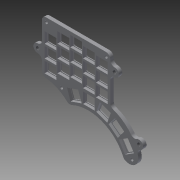
# Autodesk Inventor part: 20kb rebuild Printable Right
Saved by Autodesk Inventor 2015 SP2 (Build 190223200, 223)
## iProperties
Created: 2016-01-05
Part Number: 20kb rebuild Printable Right
Material: Generic
Document SubType Name: Modeling
Designer: Josh
Density: 1 g/cm^3
Appearance: Default
Author: Josh
Autodesk Inventor part; units mm, degrees
(part 1 of 2)
ref_plane "YZ Plane" through (0, 0, 0) normal (1, 0, 0) x (0, 1, 0)
ref_plane "XZ Plane" through (0, 0, 0) normal (0, 1, 0) x (-1, 0, 0)
ref_plane "XY Plane" through (0, 0, 0) normal (0, 0, 1) x (1, 0, 0)
sketch "Sketch1" plane through (0, 0, 0) normal (0, 0, 1) x (1, 0, 0)
  line L0 (0, 0) -> (19.05, 0)
  line L1 (19.05, 0) -> (19.05, 19.05)
  line L2 (19.05, 19.05) -> (0, 19.05)
  line L3 (0, 19.05) -> (0, 0)
  line L4 (19.05, 13.154) -> (19.05, 0)
  line L5 (19.05, 9.525) -> (38.1, 9.525)
  line L6 (38.1, 9.525) -> (38.1, 28.575)
  line L7 (38.1, 28.575) -> (19.05, 28.575)
  line L8 (19.05, 28.575) -> (19.05, 9.525)
  line L9 (38.1, 14.2875) -> (57.15, 14.2875)
  line L10 (57.15, 14.2875) -> (57.15, 33.3375)
  line L11 (57.15, 33.3375) -> (38.1, 33.3375)
  line L12 (38.1, 33.3375) -> (38.1, 14.2875)
  line L13 (57.15, 28.575) -> (76.2, 28.575)
  line L14 (76.2, 28.575) -> (76.2, 9.525)
  line L15 (76.2, 9.525) -> (57.15, 9.525)
  line L16 (57.15, 9.525) -> (57.15, 28.575)
  line L17 (76.2, 26.1938) -> (95.25, 26.1938)
  line L18 (95.25, 26.1938) -> (95.25, 7.1437)
  line L19 (95.25, 7.1437) -> (76.2, 7.1437)
  line L20 (76.2, 7.1437) -> (76.2, 26.1938)
  line L21 (19.05, 0) -> (21.4312, 0)
  line L22 (21.4312, 0) -> (21.4312, 9.525)
  line L23 (21.4312, 9.525) -> (19.05, 9.525)
  line L24 (19.05, 9.525) -> (19.05, 0)
  line L25 (38.1, 9.525) -> (40.4812, 9.525)
  line L26 (40.4812, 9.525) -> (40.4812, 14.2875)
  line L27 (40.4812, 14.2875) -> (38.1, 14.2875)
  line L28 (38.1, 14.2875) -> (38.1, 9.525)
  line L29 (57.15, 9.525) -> (54.7688, 9.525)
  line L30 (54.7688, 9.525) -> (54.7688, 14.2875)
  line L31 (54.7688, 14.2875) -> (57.15, 14.2875)
  line L32 (57.15, 14.2875) -> (57.15, 9.525)
  line L33 (76.2, 7.1437) -> (73.8187, 7.1438)
  line L34 (73.8187, 7.1438) -> (73.8187, 9.525)
  line L35 (73.8187, 9.525) -> (76.2, 9.525)
  line L36 (76.2, 9.525) -> (76.2, 7.1437)
  line L37 (39.1583, -17.1091) -> (57.15, -10.8479)
  line L38 (57.15, -10.8479) -> (50.8888, 7.1438)
  line L39 (50.8888, 7.1438) -> (32.8971, 0.8826)
  line L40 (32.8971, 0.8826) -> (39.1583, -17.1091)
  line L41 (57.15, -10.8479) -> (76.2, -10.8479)
  line L42 (76.2, -10.8479) -> (76.2, 8.2021)
  line L43 (76.2, 8.2021) -> (57.15, 8.2021)
  line L44 (57.15, 8.2021) -> (57.15, -10.8479)
  line L45 (76.2, -10.8479) -> (94.1917, -17.1091)
  line L46 (94.1917, -17.1091) -> (100.4529, 0.8826)
  line L47 (100.4529, 0.8826) -> (82.4612, 7.1437)
  line L48 (82.4612, 7.1437) -> (76.2, -10.8479)
  line L49 (94.1917, -17.1091) -> (109.1259, -28.9358)
  line L50 (109.1259, -28.9358) -> (120.9526, -14.0015)
  line L51 (120.9526, -14.0015) -> (106.0183, -2.1748)
  line L52 (106.0183, -2.1748) -> (94.1917, -17.1091)
  line L53 (109.1259, -28.9358) -> (119.3434, -45.0139)
  line L54 (119.3434, -45.0139) -> (135.4215, -34.7964)
  line L55 (135.4215, -34.7964) -> (125.204, -18.7183)
  line L56 (125.204, -18.7183) -> (109.1259, -28.9358)
  arc A0 (119.3434, -45.0139) -> (39.1583, -17.1091) centre (66.675, -67.1986) ccw
  line L57 (0, 19.05) -> (19.05, 19.05)
  line L58 (19.05, 19.05) -> (19.05, 38.1)
  line L59 (19.05, 38.1) -> (0, 38.1)
  line L60 (0, 38.1) -> (0, 19.05)
  line L61 (19.05, 28.575) -> (38.1, 28.575)
  line L62 (38.1, 28.575) -> (38.1, 47.625)
  line L63 (38.1, 47.625) -> (19.05, 47.625)
  line L64 (19.05, 47.625) -> (19.05, 28.575)
  line L65 (38.1, 33.3375) -> (57.15, 33.3375)
  line L66 (57.15, 33.3375) -> (57.15, 52.3875)
  line L67 (57.15, 52.3875) -> (38.1, 52.3875)
  line L68 (38.1, 52.3875) -> (38.1, 33.3375)
  line L69 (57.15, 47.625) -> (76.2, 47.625)
  line L70 (76.2, 47.625) -> (76.2, 28.575)
  line L71 (76.2, 28.575) -> (57.15, 28.575)
  line L72 (76.2, 45.2437) -> (95.25, 45.2437)
  line L73 (95.25, 45.2437) -> (95.25, 26.1937)
  line L74 (95.25, 26.1937) -> (76.2, 26.1937)
  line L75 (76.2, 26.1937) -> (76.2, 45.2437)
  line L76 (57.15, 33.3375) -> (57.15, 28.575)
  line L77 (0, 38.1) -> (19.05, 38.1)
  line L78 (19.05, 38.1) -> (19.05, 57.15)
  line L79 (19.05, 57.15) -> (0, 57.15)
  line L80 (0, 57.15) -> (0, 38.1)
  line L81 (19.05, 47.625) -> (38.1, 47.625)
  line L82 (38.1, 47.625) -> (38.1, 66.675)
  line L83 (38.1, 66.675) -> (19.05, 66.675)
  line L84 (19.05, 66.675) -> (19.05, 47.625)
  line L85 (38.1, 52.3875) -> (57.15, 52.3875)
  line L86 (57.15, 52.3875) -> (57.15, 71.4375)
  line L87 (57.15, 71.4375) -> (38.1, 71.4375)
  line L88 (38.1, 71.4375) -> (38.1, 52.3875)
  line L89 (57.15, 66.675) -> (76.2, 66.675)
  line L90 (76.2, 66.675) -> (76.2, 47.625)
  line L91 (76.2, 47.625) -> (57.15, 47.625)
  line L92 (76.2, 64.2938) -> (95.25, 64.2938)
  line L93 (95.25, 64.2938) -> (95.25, 45.2437)
  line L94 (95.25, 45.2437) -> (76.2, 45.2437)
  line L95 (76.2, 45.2437) -> (76.2, 64.2938)
  line L96 (57.15, 52.3875) -> (57.15, 47.625)
  line L97 (0, 71.4375) -> (9.525, 71.4375)
  line L98 (9.525, 71.4375) -> (9.525, 61.9125)
  line L99 (9.525, 61.9125) -> (0, 61.9125)
  line L100 (0, 61.9125) -> (0, 71.4375)
  line L101 (83.31, 61.9125) -> (92.835, 61.9125)
  line L102 (92.835, 61.9125) -> (92.835, 71.4375)
  line L103 (92.835, 71.4375) -> (83.31, 71.4375)
  line L104 (83.31, 71.4375) -> (83.31, 61.9125)
  line L105 (9.525, 55.5625) -> (19.05, 55.5625)
  line L106 (19.05, 55.5625) -> (19.05, 71.4375)
  line L107 (19.05, 71.4375) -> (9.525, 71.4375)
  line L108 (9.525, 71.4375) -> (9.525, 55.5625)
  circle A1 centre (7.1852, 59.8202) radius 2.0923
  line L109 (53.975, 71.4375) -> (57.15, 71.4375)
  line L110 (57.15, 71.4375) -> (57.15, 74.6125)
  line L111 (57.15, 74.6125) -> (53.975, 74.6125)
  line L112 (53.975, 74.6125) -> (53.975, 71.4375)
  line L113 (0, 0) -> (-3.175, 0)
  line L114 (-3.175, 0) -> (-3.175, -3.175)
  line L115 (-3.175, -3.175) -> (0, -3.175)
  line L116 (0, -3.175) -> (0, 0)
  line L117 (95.25, 7.1437) -> (98.425, 7.1437)
  line L118 (98.425, 7.1437) -> (98.425, 10.3187)
  line L119 (98.425, 10.3187) -> (95.25, 10.3187)
  line L120 (95.25, 10.3187) -> (95.25, 7.1437)
  line L121 (95.25, 64.2938) -> (98.425, 64.2938)
  line L122 (98.425, 64.2938) -> (98.425, 67.4688)
  line L123 (98.425, 67.4688) -> (95.25, 67.4688)
  line L124 (95.25, 67.4688) -> (95.25, 64.2938)
  line L125 (-3.175, -3.175) -> (-3.175, 74.6125)
  line L126 (-3.175, 74.6125) -> (98.425, 74.6125)
  line L127 (98.425, 74.6125) -> (98.425, 7.1437)
  line L128 (40.2019, -20.1077) -> (39.1583, -17.1091)
  line L129 (39.1583, -17.1091) -> (36.1597, -18.1526)
  line L130 (36.1597, -18.1526) -> (37.2033, -21.1512)
  line L131 (37.2033, -21.1512) -> (40.2019, -20.1077)
  line L132 (40.2019, -20.1077) -> (36.1597, -18.1526) construction
  line L133 (39.1583, -17.1091) -> (37.2033, -21.1512) construction
  line L134 (116.6637, -46.7168) -> (118.3666, -49.3965)
  line L135 (118.3666, -49.3965) -> (121.0463, -47.6936)
  line L136 (121.0463, -47.6936) -> (119.3434, -45.0139)
  line L137 (119.3434, -45.0139) -> (116.6637, -46.7168)
  line L138 (116.6637, -46.7168) -> (121.0463, -47.6936) construction
  line L139 (118.3666, -49.3965) -> (119.3434, -45.0139) construction
  line L140 (135.4215, -34.7964) -> (137.1244, -37.4761)
  line L141 (137.1244, -37.4761) -> (139.8041, -35.7732)
  line L142 (139.8041, -35.7732) -> (138.1012, -33.0935)
  line L143 (138.1012, -33.0935) -> (135.4215, -34.7964)
  line L144 (135.4215, -34.7964) -> (139.8041, -35.7732) construction
  line L145 (137.1244, -37.4761) -> (138.1012, -33.0935) construction
  arc A2 (37.2033, -21.1512) -> (-3.175, -3.175) centre (-3.175, -57.512) ccw
  arc A3 (118.3666, -49.3965) -> (37.2033, -21.1512) centre (65.4005, -70.8608) ccw
  arc A4 (118.3666, -49.3965) -> (139.8041, -35.7732) centre (126.6171, -38.7007) ccw
  arc A5 (139.8041, -35.7732) -> (98.425, 7.1437) centre (84.0124, -48.1591) ccw
  point P0 (82.4612, 26.1937)
  point P1 (82.4612, 45.2437)
  point P2 (38.1808, -19.1302)
  point P3 (118.855, -47.2052)
  point P4 (137.6128, -35.2848)
  dimension "d0" = 19.05
  dimension "d1" = 9.525
  dimension "d2" = 4.7625
  dimension "d3" = 2.3813
  dimension "d4" = 57.15
  dimension "d7" = 19.05
  dimension "d12" = 9.525
  dimension "d13" = 9.525
  dimension "d14" = 15.875
  dimension "d15" = 3.175
  constraints: 292 end point, 48 parallel, 40 equal length, 25 perpendicular, 23 collinear, 17 horizontal, 14 point on circle, 6 centre point, 6 midpoint, 4 point on line, 3 tangent, 2 equal radius, 1 coincident, 1 vertical, 83 other
  measures "d0" distance of L2.end L1.end
  measures "d1" distance of L21.end L22.end
  measures "d2" distance of L25.end L26.end
  measures "d3" distance of L33.end L34.end
  measures "d4" radius of A0
  measures "d7" distance of L1.end L59.start
  measures "d12" distance of L98.end L99.end
  measures "d13" distance of L102.end L103.end
  measures "d14" distance of L97.end L105.start
  measures "d15" distance of L111.end L110.end
extrude "Extrusion1" add sketch "Sketch1" along normal blind 5.08 contours L3 L2 L1 L0 | A1 | L113 L125 L126 L112 L87 L88 L83 L106 L107 L97 L100 L99 L108 L79 L80 L60 L3 | L116 L115 L114 L113 | L0 L21 L22 L5 L25 L26 L9 L30 L29 L15 L34 L43 L44 L38 L39 L40 L129 L130 A2 L115 L116 | L1 L5 L22 L21 | L60 L59 L58 L8 L2 | L1 L8 L7 L6 L5 | L80 L79 L108 L105 L78 L64 L59 | L58 L64 L63 L62 L12 L7 | L130 L129 L128 A3 | L111 L110 L87 L112 | L6 L9 L26 L25 | L12 L11 L10 L9 L6 | L78 L84 L83 L82 L68 L63 | L108 L98 L107 L106 L84 L79 | L79 L78 L105 L108 | L128 L37 L41 L45 L49 L53 L137 A3 | L126 L127 L123 L124 L92 L102 L103 L104 L90 L89 L86 L110 | L87 L86 L67 L82 L88 | L62 L68 L67 L66 L11 | L99 L100 L97 L98 | A0 L37 | L40 L39 L38 A0 | L137 L136 L135 A3 | L66 L69 L70 L13 L10 | A0 L41 | L44 L43 L34 L33 L42 A0 | A0 L56 L55 L54 | L53 A0 | L54 L140 L141 A4 L135 L136 | L89 L90 L69 L66 L86 | L122 L121 L124 L123 | L9 L16 L29 L30 | L13 L14 L15 L16 L10 | A0 L45 | L42 L19 L48 | L48 L47 L46 A0 | A0 L52 L51 L50 | L50 L51 L52 L46 L47 L19 L117 A5 L142 L143 L55 L56 | L49 A0 | L143 L142 L141 L140 | L127 L119 L18 L73 L93 L121 | L70 L72 L73 L17 L14 | L90 L92 L104 L101 L102 L93 L72 L70 | L20 L14 L17 L18 L19 | L33 L34 L43 L20 | L34 L15 L20 L43 | L117 L18 L119 L118 | L104 L103 L102 L92 | L92 L102 L101 L104
sketch "Sketch2" plane through (0, 0, 5.08) normal (0, 0, 1) x (1, 0, 0)
  line L0 (0, 0) -> (19.05, 0) projected
  line L1 (0, 19.05) -> (0, 0) projected
  line L2 (19.05, 19.05) -> (0, 19.05) projected
  line L3 (19.05, 0) -> (19.05, 19.05) projected
  line L4 (19.05, 9.525) -> (38.1, 9.525) projected
  line L5 (19.05, 28.575) -> (19.05, 9.525) projected
  line L6 (38.1, 9.525) -> (38.1, 28.575) projected
  line L7 (38.1, 28.575) -> (19.05, 28.575) projected
  line L8 (38.1, 14.2875) -> (57.15, 14.2875) projected
  line L9 (57.15, 33.3375) -> (38.1, 33.3375) projected
  line L10 (57.15, 14.2875) -> (57.15, 33.3375) projected
  line L11 (57.15, 28.575) -> (76.2, 28.575) projected
  line L12 (76.2, 9.525) -> (57.15, 9.525) projected
  line L13 (76.2, 26.1938) -> (95.25, 26.1938) projected
  line L14 (95.25, 26.1938) -> (95.25, 7.1437) projected
  line L15 (95.25, 7.1437) -> (76.2, 7.1437) projected
  line L16 (76.2, 28.575) -> (76.2, 9.525) projected
  line L17 (38.1, 33.3375) -> (38.1, 14.2875) projected
  line L18 (57.15, 9.525) -> (57.15, 28.575) projected
  line L19 (76.2, 7.1437) -> (76.2, 26.1938) projected
  line L20 (19.05, 19.05) -> (0, 0) construction
  line L21 (0, 19.05) -> (19.05, 0) construction
  line L22 (19.05, 28.575) -> (38.1, 9.525) construction
  line L23 (38.1, 28.575) -> (19.05, 9.525) construction
  line L24 (38.1, 33.3375) -> (57.15, 14.2875) construction
  line L25 (57.15, 33.3375) -> (38.1, 14.2875) construction
  line L26 (57.15, 28.575) -> (76.2, 9.525) construction
  line L27 (76.2, 28.575) -> (57.15, 9.525) construction
  line L28 (76.2, 26.1938) -> (95.25, 7.1437) construction
  line L29 (76.2, 7.1437) -> (95.25, 26.1938) construction
  line L30 (2.525, 2.525) -> (16.525, 2.525)
  line L31 (16.525, 2.525) -> (16.525, 16.525)
  line L32 (16.525, 16.525) -> (2.525, 16.525)
  line L33 (2.525, 16.525) -> (2.525, 2.525)
  line L34 (2.525, 2.525) -> (16.525, 16.525) construction
  line L35 (16.525, 2.525) -> (2.525, 16.525) construction
  line L36 (21.575, 12.05) -> (35.575, 12.05)
  line L37 (35.575, 12.05) -> (35.575, 26.05)
  line L38 (35.575, 26.05) -> (21.575, 26.05)
  line L39 (21.575, 26.05) -> (21.575, 12.05)
  line L40 (21.575, 12.05) -> (35.575, 26.05) construction
  line L41 (35.575, 12.05) -> (21.575, 26.05) construction
  line L42 (40.625, 16.8125) -> (54.625, 16.8125)
  line L43 (54.625, 16.8125) -> (54.625, 30.8125)
  line L44 (54.625, 30.8125) -> (40.625, 30.8125)
  line L45 (40.625, 30.8125) -> (40.625, 16.8125)
  line L46 (40.625, 16.8125) -> (54.625, 30.8125) construction
  line L47 (54.625, 16.8125) -> (40.625, 30.8125) construction
  line L48 (59.675, 12.05) -> (73.675, 12.05)
  line L49 (73.675, 12.05) -> (73.675, 26.05)
  line L50 (73.675, 26.05) -> (59.675, 26.05)
  line L51 (59.675, 26.05) -> (59.675, 12.05)
  line L52 (59.675, 12.05) -> (73.675, 26.05) construction
  line L53 (73.675, 12.05) -> (59.675, 26.05) construction
  line L54 (78.725, 9.6688) -> (92.725, 9.6688)
  line L55 (92.725, 9.6688) -> (92.725, 23.6688)
  line L56 (92.725, 23.6688) -> (78.725, 23.6688)
  line L57 (78.725, 23.6688) -> (78.725, 9.6688)
  line L58 (78.725, 9.6688) -> (92.725, 23.6688) construction
  line L59 (92.725, 9.6688) -> (78.725, 23.6688) construction
  line L60 (1.775, 3.125) -> (17.275, 3.125)
  line L61 (17.275, 3.125) -> (17.275, 15.925)
  line L62 (17.275, 15.925) -> (1.775, 15.925)
  line L63 (1.775, 15.925) -> (1.775, 3.125)
  line L64 (1.775, 3.125) -> (17.275, 15.925) construction
  line L65 (17.275, 3.125) -> (1.775, 15.925) construction
  line L66 (20.825, 12.65) -> (36.325, 12.65)
  line L67 (36.325, 12.65) -> (36.325, 25.45)
  line L68 (36.325, 25.45) -> (20.825, 25.45)
  line L69 (20.825, 25.45) -> (20.825, 12.65)
  line L70 (20.825, 12.65) -> (36.325, 25.45) construction
  line L71 (36.325, 12.65) -> (20.825, 25.45) construction
  line L72 (39.875, 17.4125) -> (55.375, 17.4125)
  line L73 (55.375, 17.4125) -> (55.375, 30.2125)
  line L74 (55.375, 30.2125) -> (39.875, 30.2125)
  line L75 (39.875, 30.2125) -> (39.875, 17.4125)
  line L76 (39.875, 17.4125) -> (55.375, 30.2125) construction
  line L77 (55.375, 17.4125) -> (39.875, 30.2125) construction
  line L78 (58.925, 12.65) -> (74.425, 12.65)
  line L79 (74.425, 12.65) -> (74.425, 25.45)
  line L80 (74.425, 25.45) -> (58.925, 25.45)
  line L81 (58.925, 25.45) -> (58.925, 12.65)
  line L82 (58.925, 12.65) -> (74.425, 25.45) construction
  line L83 (74.425, 12.65) -> (58.925, 25.45) construction
  line L84 (77.975, 10.2688) -> (93.475, 10.2688)
  line L85 (93.475, 10.2688) -> (93.475, 23.0688)
  line L86 (93.475, 23.0688) -> (77.975, 23.0688)
  line L87 (77.975, 23.0688) -> (77.975, 10.2688)
  line L88 (77.975, 10.2688) -> (93.475, 23.0688) construction
  line L89 (93.475, 10.2688) -> (77.975, 23.0688) construction
  point P0 (9.525, 9.525)
  point P1 (28.575, 19.05)
  point P2 (47.625, 23.8125)
  point P3 (66.675, 19.05)
  point P4 (85.725, 16.6687)
  dimension "d18" = 14
  dimension "d19" = 15.5
  dimension "d20" = 12.8
  constraints: 140 end point, 26 midpoint, 21 parallel, 18 perpendicular, 17 equal length, 10 horizontal
  measures "d18" distance of L31.end L32.end
  measures "d19" distance of L61.end L62.end
  measures "d20" distance of L60.end L61.end
extrude "Extrusion2" cut sketch "Sketch2" against normal blind 5.08 contours L33 L60 L31 L30 | L60 L63 L62 L33 | L33 L62 L31 L60 | L31 L62 L61 L60 | L33 L32 L31 L62 | L39 L66 L37 L36 | L66 L69 L68 L39 | L39 L68 L37 L66 | L37 L68 L67 L66 | L39 L38 L37 L68 | L45 L72 L43 L42 | L72 L75 L74 L45 | L45 L74 L43 L72 | L43 L74 L73 L72 | L45 L44 L43 L74 | L51 L78 L49 L48 | L78 L81 L80 L51 | L51 L80 L49 L78 | L49 L80 L79 L78 | L51 L50 L49 L80 | L57 L84 L55 L54 | L84 L87 L86 L57 | L57 L86 L55 L84 | L55 L86 L85 L84 | L57 L56 L55 L86
sketch "Sketch3" plane through (0, 0, 5.08) normal (0, 0, 1) x (1, 0, 0)
  line L0 (0.775, 1.525) -> (18.275, 1.525)
  line L1 (18.275, 1.525) -> (18.275, 17.525)
  line L2 (18.275, 17.525) -> (0.775, 17.525)
  line L3 (0.775, 17.525) -> (0.775, 1.525)
  line L4 (0.775, 1.525) -> (18.275, 17.525) construction
  line L5 (18.275, 1.525) -> (0.775, 17.525) construction
  line L6 (19.825, 27.05) -> (37.325, 27.05)
  line L7 (37.325, 27.05) -> (37.325, 11.05)
  line L8 (37.325, 11.05) -> (19.825, 11.05)
  line L9 (19.825, 11.05) -> (19.825, 27.05)
  line L10 (19.825, 27.05) -> (37.325, 11.05) construction
  line L11 (37.325, 27.05) -> (19.825, 11.05) construction
  line L12 (38.875, 31.8125) -> (56.375, 31.8125)
  line L13 (56.375, 31.8125) -> (56.375, 15.8125)
  line L14 (56.375, 15.8125) -> (38.875, 15.8125)
  line L15 (38.875, 15.8125) -> (38.875, 31.8125)
  line L16 (38.875, 31.8125) -> (56.375, 15.8125) construction
  line L17 (56.375, 31.8125) -> (38.875, 15.8125) construction
  line L18 (75.425, 27.05) -> (57.925, 27.05)
  line L19 (57.925, 27.05) -> (57.925, 11.05)
  line L20 (57.925, 11.05) -> (75.425, 11.05)
  line L21 (75.425, 11.05) -> (75.425, 27.05)
  line L22 (75.425, 27.05) -> (57.925, 11.05) construction
  line L23 (57.925, 27.05) -> (75.425, 11.05) construction
  line L24 (76.975, 8.6687) -> (94.475, 8.6687)
  line L25 (94.475, 8.6687) -> (94.475, 24.6687)
  line L26 (94.475, 24.6687) -> (76.975, 24.6687)
  line L27 (76.975, 24.6687) -> (76.975, 8.6687)
  line L28 (76.975, 8.6687) -> (94.475, 24.6687) construction
  line L29 (94.475, 8.6687) -> (76.975, 24.6687) construction
  point P0 (0, 0)
  point P1 (9.525, 9.525)
  point P2 (28.575, 19.05)
  point P3 (47.625, 23.8125)
  point P4 (66.675, 19.05)
  point P5 (85.725, 16.6687)
  dimension "d23" = 17.5
  dimension "d24" = 16
  constraints: 60 end point, 17 parallel, 10 midpoint, 5 horizontal, 5 perpendicular, 1 point on line
  measures "d23" distance of L1.end L2.end
  measures "d24" distance of L0.end L1.end
extrude "Extrusion3" cut sketch "Sketch3" against normal blind 3.98
pattern_linear "Rectangular Pattern1" count 3 spacing 19.05 along (0, 1, 0) of "Extrusion2", "Extrusion3"
sketch "Sketch4" plane through (0, 0, 5.08) normal (0, 0, 1) x (1, 0, 0)
  line L0 (57.15, -10.8479) -> (50.8888, 7.1438) projected
  line L1 (39.1583, -17.1091) -> (57.15, -10.8479) projected
  line L2 (32.8971, 0.8826) -> (39.1583, -17.1091) projected
  line L3 (50.8888, 7.1438) -> (32.8971, 0.8826) projected
  line L4 (57.15, 8.2021) -> (57.15, -10.8479) projected
  line L5 (76.2, 8.2021) -> (57.15, 8.2021) projected
  line L6 (76.2, -10.8479) -> (76.2, 8.2021) projected
  line L7 (57.15, -10.8479) -> (76.2, -10.8479) projected
  line L8 (82.4612, 7.1437) -> (76.2, -10.8479) projected
  line L9 (100.4529, 0.8826) -> (82.4612, 7.1437) projected
  line L10 (94.1917, -17.1091) -> (100.4529, 0.8826) projected
  line L11 (76.2, -10.8479) -> (94.1917, -17.1091) projected
  line L12 (106.0183, -2.1748) -> (94.1917, -17.1091) projected
  line L13 (120.9526, -14.0015) -> (106.0183, -2.1748) projected
  line L14 (109.1259, -28.9358) -> (120.9526, -14.0015) projected
  line L15 (94.1917, -17.1091) -> (109.1259, -28.9358) projected
  line L16 (109.1259, -28.9358) -> (119.3434, -45.0139) projected
  line L17 (125.204, -18.7183) -> (109.1259, -28.9358) projected
  line L18 (135.4215, -34.7964) -> (125.204, -18.7183) projected
  line L19 (119.3434, -45.0139) -> (135.4215, -34.7964) projected
  line L20 (32.8971, 0.8826) -> (57.15, -10.8479) construction
  line L21 (50.8888, 7.1438) -> (39.1583, -17.1091) construction
  line L22 (57.15, 8.2021) -> (76.2, -10.8479) construction
  line L23 (76.2, 8.2021) -> (57.15, -10.8479) construction
  line L24 (82.4612, 7.1437) -> (94.1917, -17.1091) construction
  line L25 (76.2, -10.8479) -> (100.4529, 0.8826) construction
  line L26 (106.0183, -2.1748) -> (109.1259, -28.9358) construction
  line L27 (120.9526, -14.0015) -> (94.1917, -17.1091) construction
  line L28 (125.204, -18.7183) -> (119.3434, -45.0139) construction
  line L29 (109.1259, -28.9358) -> (135.4215, -34.7964) construction
  line L30 (-25.4225, -31.5333) -> (-11.4225, -31.5333) construction
  line L31 (-11.4225, -31.5333) -> (-11.4225, -17.5333) construction
  line L32 (-11.4225, -17.5333) -> (-25.4225, -17.5333) construction
  line L33 (-25.4225, -17.5333) -> (-25.4225, -31.5333) construction
  line L34 (-25.4225, -31.5333) -> (-11.4225, -17.5333) construction
  line L35 (-11.4225, -31.5333) -> (-25.4225, -17.5333) construction
  line L36 (-21.2907, -27.4015) -> (-15.5542, -27.4015) construction
  line L37 (-15.5542, -27.4015) -> (-15.5542, -21.6651) construction
  line L38 (-15.5542, -21.6651) -> (-21.2907, -21.6651) construction
  line L39 (-21.2907, -21.6651) -> (-21.2907, -27.4015) construction
  line L40 (-21.2907, -27.4015) -> (-15.5542, -21.6651) construction
  line L41 (-15.5542, -27.4015) -> (-21.2907, -21.6651) construction
  line L42 (79.4146, -9.2931) -> (92.6368, -13.8945)
  line L43 (92.6368, -13.8945) -> (97.2382, -0.6723)
  line L44 (97.2382, -0.6723) -> (84.016, 3.9291)
  line L45 (84.016, 3.9291) -> (79.4146, -9.2931)
  line L46 (79.4146, -9.2931) -> (97.2382, -0.6723) construction
  line L47 (92.6368, -13.8945) -> (84.016, 3.9291) construction
  line L48 (97.7387, -16.6972) -> (108.714, -25.3887)
  line L49 (108.714, -25.3887) -> (117.4056, -14.4134)
  line L50 (117.4056, -14.4134) -> (106.4302, -5.7219)
  line L51 (106.4302, -5.7219) -> (97.7387, -16.6972)
  line L52 (97.7387, -16.6972) -> (117.4056, -14.4134) construction
  line L53 (108.714, -25.3887) -> (106.4302, -5.7219) construction
  line L54 (112.6113, -29.7126) -> (120.1202, -41.5285)
  line L55 (120.1202, -41.5285) -> (131.9361, -34.0196)
  line L56 (131.9361, -34.0196) -> (124.4272, -22.2037)
  line L57 (124.4272, -22.2037) -> (112.6113, -29.7126)
  line L58 (112.6113, -29.7126) -> (131.9361, -34.0196) construction
  line L59 (120.1202, -41.5285) -> (124.4272, -22.2037) construction
  line L60 (40.7132, -13.8945) -> (53.9354, -9.2931)
  line L61 (53.9354, -9.2931) -> (49.334, 3.9291)
  line L62 (49.334, 3.9291) -> (36.1118, -0.6723)
  line L63 (36.1118, -0.6723) -> (40.7132, -13.8945)
  line L64 (40.7132, -13.8945) -> (49.334, 3.9291) construction
  line L65 (53.9354, -9.2931) -> (36.1118, -0.6723) construction
  line L66 (59.675, -8.3229) -> (73.675, -8.3229)
  line L67 (73.675, -8.3229) -> (73.675, 5.6771)
  line L68 (73.675, 5.6771) -> (59.675, 5.6771)
  line L69 (59.675, 5.6771) -> (59.675, -8.3229)
  line L70 (59.675, -8.3229) -> (73.675, 5.6771) construction
  line L71 (73.675, -8.3229) -> (59.675, 5.6771) construction
  line L72 (35.6006, -1.4854) -> (50.2395, 3.609)
  line L73 (50.2395, 3.609) -> (54.4465, -8.4799)
  line L74 (54.4465, -8.4799) -> (39.8076, -13.5743)
  line L75 (39.8076, -13.5743) -> (35.6006, -1.4854)
  line L76 (35.6006, -1.4854) -> (54.4465, -8.4799) construction
  line L77 (50.2395, 3.609) -> (39.8076, -13.5743) construction
  line L78 (58.925, -7.7229) -> (74.425, -7.7229)
  line L79 (74.425, -7.7229) -> (74.425, 5.0771)
  line L80 (74.425, 5.0771) -> (58.925, 5.0771)
  line L81 (58.925, 5.0771) -> (58.925, -7.7229)
  line L82 (58.925, -7.7229) -> (74.425, 5.0771) construction
  line L83 (74.425, -7.7229) -> (58.925, 5.0771) construction
  line L84 (121.0289, -41.8397) -> (112.7154, -28.7578)
  line L85 (112.7154, -28.7578) -> (123.5186, -21.8925)
  line L86 (123.5186, -21.8925) -> (131.832, -34.9744)
  line L87 (131.832, -34.9744) -> (121.0289, -41.8397)
  line L88 (121.0289, -41.8397) -> (123.5186, -21.8925) construction
  line L89 (112.7154, -28.7578) -> (131.832, -34.9744) construction
  line L90 (-26.1725, -18.1333) -> (-10.6725, -18.1333) construction
  line L91 (-10.6725, -18.1333) -> (-10.6725, -30.9333) construction
  line L92 (-10.6725, -30.9333) -> (-26.1725, -30.9333) construction
  line L93 (-26.1725, -30.9333) -> (-26.1725, -18.1333) construction
  line L94 (-26.1725, -18.1333) -> (-10.6725, -30.9333) construction
  line L95 (-10.6725, -18.1333) -> (-26.1725, -30.9333) construction
  line L96 (97.5233, -15.7612) -> (109.6745, -25.384)
  line L97 (109.6745, -25.384) -> (117.621, -15.3494)
  line L98 (117.621, -15.3494) -> (105.4698, -5.7266)
  line L99 (105.4698, -5.7266) -> (97.5233, -15.7612)
  line L100 (97.5233, -15.7612) -> (117.621, -15.3494) construction
  line L101 (109.6745, -25.384) -> (105.4698, -5.7266) construction
  line L102 (78.9035, -8.4799) -> (93.5424, -13.5743)
  line L103 (93.5424, -13.5743) -> (97.7494, -1.4854)
  line L104 (97.7494, -1.4854) -> (83.1105, 3.609)
  line L105 (83.1105, 3.609) -> (78.9035, -8.4799)
  line L106 (78.9035, -8.4799) -> (97.7494, -1.4854) construction
  line L107 (93.5424, -13.5743) -> (83.1105, 3.609) construction
  point P0 (0, 0)
  point P1 (-18.4225, -24.5333)
  point P2 (-18.4225, -24.5333)
  point P3 (88.3264, -4.9827)
  point P4 (107.5721, -15.5553)
  point P5 (122.2737, -31.8661)
  point P6 (45.0236, -4.9827)
  point P7 (66.675, -1.3229)
  dimension "d30" = 14
  dimension "d31" = 15.5
  dimension "d32" = 12.8
  constraints: 176 end point, 36 parallel, 32 midpoint, 21 equal length, 18 perpendicular, 3 horizontal, 1 point on line
  measures "d30" distance of L31.end L32.end
  measures "d31" distance of L90.start L90.end
  measures "d32" distance of L90.end L91.end
extrude "Extrusion4" cut sketch "Sketch4" against normal blind 5.08 contours L45 L102 L43 L42 | L102 L105 L104 L45 | L45 L104 L43 L102 | L43 L104 L103 L102 | L45 L44 L43 L104 | L51 L96 L49 L48 | L96 L99 L98 L51 | L51 L98 L49 L96 | L49 L98 L97 L96 | L51 L50 L49 L98 | L57 L84 L55 L54 | L84 L85 L86 L57 | L57 L86 L55 L84 | L55 L86 L87 L84 | L57 L56 L55 L86 | L63 L74 L61 L60 | L74 L75 L72 L63 | L63 L72 L61 L74 | L61 L72 L73 L74 | L63 L62 L61 L72 | L69 L78 L67 L66 | L78 L81 L80 L69 | L69 L80 L67 L78 | L67 L80 L79 L78 | L69 L68 L67 L80
sketch "Sketch5" plane through (0, 0, 5.08) normal (0, 0, 1) x (1, 0, 0)
  line L0 (18.275, 1.525) -> (0.775, 1.525) projected
  line L1 (18.275, 17.525) -> (18.275, 1.525) projected
  line L2 (0.775, 17.525) -> (18.275, 17.525) projected
  line L3 (0.775, 1.525) -> (0.775, 17.525) projected
  line L4 (53.9354, -9.2931) -> (40.7132, -13.8945) projected
  line L5 (73.675, -8.3229) -> (59.675, -8.3229) projected
  line L6 (92.6368, -13.8945) -> (79.4146, -9.2931) projected
  line L7 (108.714, -25.3887) -> (97.7387, -16.6972) projected
  line L8 (120.1202, -41.5285) -> (112.6113, -29.7126) projected
  line L9 (39.3891, -15.4141) -> (55.9168, -9.6624)
  line L10 (55.9168, -9.6624) -> (50.6581, 5.4488)
  line L11 (50.6581, 5.4488) -> (34.1303, -0.303)
  line L12 (34.1303, -0.303) -> (39.3891, -15.4141)
  line L13 (39.3891, -15.4141) -> (50.6581, 5.4488) construction
  line L14 (55.9168, -9.6624) -> (34.1303, -0.303) construction
  line L15 (57.925, -9.3229) -> (75.425, -9.3229)
  line L16 (75.425, -9.3229) -> (75.425, 6.6771)
  line L17 (75.425, 6.6771) -> (57.925, 6.6771)
  line L18 (57.925, 6.6771) -> (57.925, -9.3229)
  line L19 (57.925, -9.3229) -> (75.425, 6.6771) construction
  line L20 (75.425, -9.3229) -> (57.925, 6.6771) construction
  line L21 (77.4332, -9.6624) -> (93.9609, -15.4141)
  line L22 (93.9609, -15.4141) -> (99.2197, -0.303)
  line L23 (99.2197, -0.303) -> (82.6919, 5.4488)
  line L24 (82.6919, 5.4488) -> (77.4332, -9.6624)
  line L25 (77.4332, -9.6624) -> (99.2197, -0.303) construction
  line L26 (93.9609, -15.4141) -> (82.6919, 5.4488) construction
  line L27 (109.4651, -27.2591) -> (95.746, -16.3947)
  line L28 (95.746, -16.3947) -> (105.6792, -3.8515)
  line L29 (105.6792, -3.8515) -> (119.3983, -14.7159)
  line L30 (119.3983, -14.7159) -> (109.4651, -27.2591)
  line L31 (109.4651, -27.2591) -> (105.6792, -3.8515) construction
  line L32 (95.746, -16.3947) -> (119.3983, -14.7159) construction
  line L33 (120.2148, -43.5419) -> (110.8287, -28.7719)
  line L34 (110.8287, -28.7719) -> (124.3326, -20.1903)
  line L35 (124.3326, -20.1903) -> (133.7188, -34.9602)
  line L36 (133.7188, -34.9602) -> (120.2148, -43.5419)
  line L37 (120.2148, -43.5419) -> (124.3326, -20.1903) construction
  line L38 (110.8287, -28.7719) -> (133.7188, -34.9602) construction
  point P0 (0, 0)
  point P1 (45.0236, -4.9827)
  point P2 (66.675, -1.3229)
  point P3 (88.3264, -4.9827)
  point P4 (107.5721, -15.5553)
  point P5 (122.2737, -31.8661)
  constraints: 60 end point, 15 parallel, 10 equal length, 10 midpoint, 5 perpendicular
extrude "Extrusion5" cut sketch "Sketch5" against normal blind 3.98 contours L12 L11 L10 L9 | L18 L17 L16 L15 | L24 L23 L22 L21 | L27 L28 L29 L30 | L33 L34 L35 L36
fillet "Fillet1" radius 6.35 6 edges at (37.2033, -21.1512, 2.54) (-3.175, -3.175, 2.54) (98.425, 7.1438, 2.54) (98.425, 74.6125, 2.54) (-3.175, 74.6125, 2.54) (118.3666, -49.3965, 2.54)
sketch "Sketch6" plane through (0, 0, 0) normal (0, 0, -1) x (-1, 0, 0)
  line L0 (-37.9981, 73.8371) -> (-5.6484, 73.8371) construction
  line L1 (-5.6484, 73.8371) -> (-5.6484, 68.2625) construction
  line L2 (-5.6484, 68.2625) -> (-37.9981, 68.2625) construction
  line L3 (-37.9981, 68.2625) -> (-37.9981, 73.8371) construction
  line L4 (-89.6016, 73.8371) -> (-70.2241, 73.8371) construction
  line L5 (-70.2241, 73.8371) -> (-70.2241, 68.2625) construction
  line L6 (-70.2241, 68.2625) -> (-89.6016, 68.2625) construction
  line L7 (-89.6016, 68.2625) -> (-89.6016, 73.8371) construction
  line L8 (-114.209, 73.8371) -> (51.1131, 73.8371) construction
  line L9 (-70.2241, 68.2625) -> (-37.9981, 68.2625) construction
  line L10 (-37.9981, 68.2625) -> (-37.9981, 73.8371) construction
  line L11 (-37.9981, 73.8371) -> (-70.2241, 73.8371) construction
  line L12 (-70.2241, 73.8371) -> (-70.2241, 68.2625) construction
  arc A0 (-92.075, 74.6125) -> (-98.425, 68.2625) centre (-92.075, 68.2625) ccw construction
  arc A1 (3.175, 68.2625) -> (-3.175, 74.6125) centre (-3.175, 68.2625) ccw construction
  line L13 (-3.175, 68.2625) -> (-5.6484, 68.2625) construction
  line L14 (-92.075, 68.2625) -> (-89.6016, 68.2625) construction
  line L15 (-35.4664, 70.6533) -> (-35.9925, 70.6533)
  line L16 (-35.9925, 70.6533) -> (-37.1065, 72.0711)
  line L17 (-37.1065, 72.0711) -> (-37.2843, 71.871)
  line L18 (-37.2843, 71.871) -> (-37.2843, 70.6533)
  line L19 (-37.2843, 70.6533) -> (-37.6894, 70.6533)
  line L20 (-37.6894, 70.6533) -> (-37.6894, 73.7013)
  line L21 (-37.6894, 73.7013) -> (-37.2843, 73.7013)
  line L22 (-37.2843, 73.7013) -> (-37.2843, 72.3008)
  line L23 (-37.2843, 72.3008) -> (-36.0345, 73.7013)
  line L24 (-36.0345, 73.7013) -> (-35.5405, 73.7013)
  line L25 (-35.5405, 73.7013) -> (-36.8026, 72.3403)
  line L26 (-36.8026, 72.3403) -> (-35.4664, 70.6533)
  spline S0 degree 2 poles (-34.261, 70.6014) (-34.8093, 70.6014) (-35.412, 71.2165) (-35.412, 71.7846) knots 0 0 0 1 2 2 2
  spline S1 degree 2 poles (-35.412, 71.7846) (-35.412, 72.3428) (-34.8266, 73.0047) (-34.3549, 73.0047) knots 0 0 0 1 2 2 2
  spline S2 degree 2 poles (-34.3549, 73.0047) (-34.1424, 73.0047) (-33.8139, 72.8812) (-33.6929, 72.7503) knots 0 0 0 1 2 2 2
  spline S3 degree 2 poles (-33.6929, 72.7503) (-33.5694, 72.6194) (-33.4385, 72.2415) (-33.4385, 71.9673) knots 0 0 0 1 2 2 2
  line L27 (-33.4385, 71.9673) -> (-33.4385, 71.7574)
  line L28 (-33.4385, 71.7574) -> (-35.0218, 71.7574)
  spline S4 degree 2 poles (-35.0218, 71.7574) (-35.0218, 71.3597) (-34.6216, 70.9373) (-34.2659, 70.9373) knots 0 0 0 1 2 2 2
  spline S5 degree 2 poles (-34.2659, 70.9373) (-34.14, 70.9373) (-33.8954, 70.9941) (-33.7966, 71.0386) knots 0 0 0 1 2 2 2
  spline S6 degree 2 poles (-33.7966, 71.0386) (-33.6929, 71.088) (-33.5496, 71.1745) (-33.5027, 71.214) knots 0 0 0 1 2 2 2
  line L29 (-33.5027, 71.214) -> (-33.4805, 71.214)
  line L30 (-33.4805, 71.214) -> (-33.4805, 70.7941)
  spline S7 degree 2 poles (-33.4805, 70.7941) (-33.5472, 70.7669) (-33.7497, 70.6879) (-33.8287, 70.6656) knots 0 0 0 1 2 2 2
  spline S8 degree 2 poles (-33.8287, 70.6656) (-33.9399, 70.6335) (-34.1227, 70.6014) (-34.261, 70.6014) knots 0 0 0 1 2 2 2
  spline S9 degree 2 poles (-33.8139, 72.0513) (-33.8189, 72.2069) (-33.8831, 72.4342) (-33.9448, 72.5107) knots 0 0 0 1 2 2 2
  spline S10 degree 2 poles (-33.9448, 72.5107) (-34.0115, 72.5972) (-34.2215, 72.6886) (-34.3771, 72.6886) knots 0 0 0 1 2 2 2
  spline S11 degree 2 poles (-34.3771, 72.6886) (-34.5302, 72.6886) (-34.7451, 72.5972) (-34.834, 72.5083) knots 0 0 0 1 2 2 2
  spline S12 degree 2 poles (-34.834, 72.5083) (-34.9205, 72.4169) (-35.0094, 72.197) (-35.0218, 72.0513) knots 0 0 0 1 2 2 2
  line L31 (-35.0218, 72.0513) -> (-33.8139, 72.0513)
  line L32 (-31.2525, 72.9405) -> (-32.4826, 69.811)
  line L33 (-32.4826, 69.811) -> (-32.8951, 69.811)
  line L34 (-32.8951, 69.811) -> (-32.4851, 70.7644)
  line L35 (-32.4851, 70.7644) -> (-33.315, 72.9405)
  line L36 (-33.315, 72.9405) -> (-32.9, 72.9405)
  line L37 (-32.9, 72.9405) -> (-32.2751, 71.2461)
  line L38 (-32.2751, 71.2461) -> (-31.6527, 72.9405)
  line L39 (-31.6527, 72.9405) -> (-31.2525, 72.9405)
  spline S13 degree 2 poles (-29.0443, 71.834) (-29.0443, 71.2733) (-29.5877, 70.5891) (-29.9978, 70.5891) knots 0 0 0 1 2 2 2
  spline S14 degree 2 poles (-29.9978, 70.5891) (-30.183, 70.5891) (-30.4473, 70.6805) (-30.5757, 70.7595) knots 0 0 0 1 2 2 2
  line L40 (-30.5757, 70.7595) -> (-30.6004, 70.6533)
  line L41 (-30.6004, 70.6533) -> (-30.9611, 70.6533)
  line L42 (-30.9611, 70.6533) -> (-30.9611, 73.8371)
  line L43 (-30.9611, 73.8371) -> (-30.5757, 73.8371)
  line L44 (-30.5757, 73.8371) -> (-30.5757, 72.7009)
  spline S15 degree 2 poles (-30.5757, 72.7009) (-30.43, 72.8318) (-30.0916, 73.0047) (-29.8767, 73.0047) knots 0 0 0 1 2 2 2
  spline S16 degree 2 poles (-29.8767, 73.0047) (-29.4889, 73.0047) (-29.0443, 72.3848) (-29.0443, 71.834) knots 0 0 0 1 2 2 2
  spline S17 degree 2 poles (-29.442, 71.8043) (-29.442, 72.2143) (-29.6915, 72.6392) (-29.9681, 72.6392) knots 0 0 0 1 2 2 2
  spline S18 degree 2 poles (-29.9681, 72.6392) (-30.1237, 72.6392) (-30.4448, 72.491) (-30.5757, 72.3774) knots 0 0 0 1 2 2 2
  line L45 (-30.5757, 72.3774) -> (-30.5757, 71.0658)
  spline S19 degree 2 poles (-30.5757, 71.0658) (-30.43, 70.9941) (-30.2052, 70.9349) (-30.0719, 70.9349) knots 0 0 0 1 2 2 2
  spline S20 degree 2 poles (-30.0719, 70.9349) (-29.7779, 70.9349) (-29.442, 71.3523) (-29.442, 71.8043) knots 0 0 0 1 2 2 2
  spline S21 degree 2 poles (-26.7645, 71.7969) (-26.7645, 71.2189) (-27.3203, 70.5891) (-27.7846, 70.5891) knots 0 0 0 1 2 2 2
  spline S22 degree 2 poles (-27.7846, 70.5891) (-28.2613, 70.5891) (-28.8072, 71.2387) (-28.8072, 71.7969) knots 0 0 0 1 2 2 2
  spline S23 degree 2 poles (-28.8072, 71.7969) (-28.8072, 72.3699) (-28.244, 73.0047) (-27.7846, 73.0047) knots 0 0 0 1 2 2 2
  spline S24 degree 2 poles (-27.7846, 73.0047) (-27.3203, 73.0047) (-26.7645, 72.3724) (-26.7645, 71.7969) knots 0 0 0 1 2 2 2
  spline S25 degree 2 poles (-27.1622, 71.7969) (-27.1622, 72.2415) (-27.4857, 72.6738) (-27.7846, 72.6738) knots 0 0 0 1 2 2 2
  spline S26 degree 2 poles (-27.7846, 72.6738) (-28.0835, 72.6738) (-28.4095, 72.2415) (-28.4095, 71.7969) knots 0 0 0 1 2 2 2
  spline S27 degree 2 poles (-28.4095, 71.7969) (-28.4095, 71.3647) (-28.0835, 70.92) (-27.7846, 70.92) knots 0 0 0 1 2 2 2
  spline S28 degree 2 poles (-27.7846, 70.92) (-27.4882, 70.92) (-27.1622, 71.3572) (-27.1622, 71.7969) knots 0 0 0 1 2 2 2
  spline S29 degree 2 poles (-25.0948, 70.8953) (-25.1417, 70.8608) (-25.2998, 70.7373) (-25.3739, 70.7002) knots 0 0 0 1 2 2 2
  spline S30 degree 2 poles (-25.3739, 70.7002) (-25.4752, 70.6459) (-25.6653, 70.5891) (-25.8382, 70.5891) knots 0 0 0 1 2 2 2
  spline S31 degree 2 poles (-25.8382, 70.5891) (-25.979, 70.5891) (-26.2334, 70.6953) (-26.3298, 70.7916) knots 0 0 0 1 2 2 2
  spline S32 degree 2 poles (-26.3298, 70.7916) (-26.4212, 70.8855) (-26.5323, 71.1621) (-26.5323, 71.3153) knots 0 0 0 1 2 2 2
  spline S33 degree 2 poles (-26.5323, 71.3153) (-26.5323, 71.5524) (-26.3322, 71.8883) (-26.1149, 71.9846) knots 0 0 0 1 2 2 2
  spline S34 degree 2 poles (-26.1149, 71.9846) (-25.9222, 72.0735) (-25.3986, 72.1402) (-25.0948, 72.1575) knots 0 0 0 1 2 2 2
  line L46 (-25.0948, 72.1575) -> (-25.0948, 72.2316)
  spline S35 degree 2 poles (-25.0948, 72.2316) (-25.0948, 72.365) (-25.1763, 72.5305) (-25.2504, 72.5774) knots 0 0 0 1 2 2 2
  spline S36 degree 2 poles (-25.2504, 72.5774) (-25.3245, 72.6244) (-25.5369, 72.654) (-25.6505, 72.654) knots 0 0 0 1 2 2 2
  spline S37 degree 2 poles (-25.6505, 72.654) (-25.7839, 72.654) (-26.1445, 72.575) (-26.3248, 72.4984) knots 0 0 0 1 2 2 2
  line L47 (-26.3248, 72.4984) -> (-26.3471, 72.4984)
  line L48 (-26.3471, 72.4984) -> (-26.3471, 72.8911)
  spline S38 degree 2 poles (-26.3471, 72.8911) (-26.2409, 72.9208) (-25.8432, 72.9949) (-25.6481, 72.9949) knots 0 0 0 1 2 2 2
  spline S39 degree 2 poles (-25.6481, 72.9949) (-25.4109, 72.9949) (-25.0874, 72.9208) (-24.9589, 72.8244) knots 0 0 0 1 2 2 2
  spline S40 degree 2 poles (-24.9589, 72.8244) (-24.8329, 72.7306) (-24.7094, 72.4317) (-24.7094, 72.2168) knots 0 0 0 1 2 2 2
  line L49 (-24.7094, 72.2168) -> (-24.7094, 70.6533)
  line L50 (-24.7094, 70.6533) -> (-25.0948, 70.6533)
  line L51 (-25.0948, 70.6533) -> (-25.0948, 70.8953)
  line L52 (-25.0948, 71.2165) -> (-25.0948, 71.8512)
  spline S41 degree 2 poles (-25.0948, 71.8512) (-25.2331, 71.8389) (-25.6505, 71.7969) (-25.7814, 71.7574) knots 0 0 0 1 2 2 2
  spline S42 degree 2 poles (-25.7814, 71.7574) (-25.9346, 71.7105) (-26.1346, 71.5153) (-26.1346, 71.3424) knots 0 0 0 1 2 2 2
  spline S43 degree 2 poles (-26.1346, 71.3424) (-26.1346, 71.1448) (-25.9123, 70.9447) (-25.6999, 70.9447) knots 0 0 0 1 2 2 2
  spline S44 degree 2 poles (-25.6999, 70.9447) (-25.5196, 70.9447) (-25.2232, 71.1004) (-25.0948, 71.2165) knots 0 0 0 1 2 2 2
  line L53 (-22.9557, 72.528) -> (-22.9755, 72.528)
  spline S45 degree 2 poles (-22.9755, 72.528) (-23.02, 72.5404) (-23.1163, 72.5453) (-23.183, 72.5453) knots 0 0 0 1 2 2 2
  spline S46 degree 2 poles (-23.183, 72.5453) (-23.3386, 72.5453) (-23.6449, 72.4095) (-23.7832, 72.2761) knots 0 0 0 1 2 2 2
  line L54 (-23.7832, 72.2761) -> (-23.7832, 70.6533)
  line L55 (-23.7832, 70.6533) -> (-24.1685, 70.6533)
  line L56 (-24.1685, 70.6533) -> (-24.1685, 72.9405)
  line L57 (-24.1685, 72.9405) -> (-23.7832, 72.9405)
  line L58 (-23.7832, 72.9405) -> (-23.7832, 72.5997)
  spline S47 degree 2 poles (-23.7832, 72.5997) (-23.5732, 72.7874) (-23.2595, 72.9405) (-23.1113, 72.9405) knots 0 0 0 1 2 2 2
  spline S48 degree 2 poles (-23.1113, 72.9405) (-23.0521, 72.9405) (-22.9928, 72.9356) (-22.9557, 72.9282) knots 0 0 0 1 2 2 2
  line L59 (-22.9557, 72.9282) -> (-22.9557, 72.528)
  line L60 (-20.8982, 70.6533) -> (-21.2835, 70.6533)
  line L61 (-21.2835, 70.6533) -> (-21.2835, 70.8855)
  spline S49 degree 2 poles (-21.2835, 70.8855) (-21.3725, 70.8114) (-21.5034, 70.7126) (-21.5923, 70.6706) knots 0 0 0 1 2 2 2
  spline S50 degree 2 poles (-21.5923, 70.6706) (-21.6738, 70.6311) (-21.8492, 70.5891) (-21.9653, 70.5891) knots 0 0 0 1 2 2 2
  spline S51 degree 2 poles (-21.9653, 70.5891) (-22.153, 70.5891) (-22.4691, 70.7447) (-22.5803, 70.8953) knots 0 0 0 1 2 2 2
  spline S52 degree 2 poles (-22.5803, 70.8953) (-22.6914, 71.046) (-22.8149, 71.4906) (-22.8149, 71.7796) knots 0 0 0 1 2 2 2
  spline S53 degree 2 poles (-22.8149, 71.7796) (-22.8149, 72.081) (-22.6593, 72.5206) (-22.5235, 72.6861) knots 0 0 0 1 2 2 2
  spline S54 degree 2 poles (-22.5235, 72.6861) (-22.3975, 72.8343) (-22.0443, 73.0047) (-21.8492, 73.0047) knots 0 0 0 1 2 2 2
  spline S55 degree 2 poles (-21.8492, 73.0047) (-21.6787, 73.0047) (-21.4243, 72.9282) (-21.2835, 72.8491) knots 0 0 0 1 2 2 2
  line L62 (-21.2835, 72.8491) -> (-21.2835, 73.8371)
  line L63 (-21.2835, 73.8371) -> (-20.8982, 73.8371)
  line L64 (-20.8982, 73.8371) -> (-20.8982, 70.6533)
  line L65 (-21.2835, 71.209) -> (-21.2835, 72.5305)
  spline S56 degree 2 poles (-21.2835, 72.5305) (-21.4268, 72.5997) (-21.654, 72.6515) (-21.7849, 72.6515) knots 0 0 0 1 2 2 2
  spline S57 degree 2 poles (-21.7849, 72.6515) (-22.0814, 72.6515) (-22.4173, 72.2069) (-22.4173, 71.787) knots 0 0 0 1 2 2 2
  spline S58 degree 2 poles (-22.4173, 71.787) (-22.4173, 71.3819) (-22.1604, 70.9546) (-21.8763, 70.9546) knots 0 0 0 1 2 2 2
  spline S59 degree 2 poles (-21.8763, 70.9546) (-21.7257, 70.9546) (-21.4194, 71.093) (-21.2835, 71.209) knots 0 0 0 1 2 2 2
  spline S60 degree 2 poles (-17.9367, 70.5891) (-18.2059, 70.5891) (-18.606, 70.7299) (-18.7468, 70.8706) knots 0 0 0 1 2 2 2
  spline S61 degree 2 poles (-18.7468, 70.8706) (-18.9074, 71.0287) (-19.0383, 71.4733) (-19.0383, 71.7994) knots 0 0 0 1 2 2 2
  line L66 (-19.0383, 71.7994) -> (-19.0383, 73.7013)
  line L67 (-19.0383, 73.7013) -> (-18.6332, 73.7013)
  line L68 (-18.6332, 73.7013) -> (-18.6332, 71.7994)
  spline S62 degree 2 poles (-18.6332, 71.7994) (-18.6332, 71.587) (-18.5789, 71.3004) (-18.5023, 71.1843) knots 0 0 0 1 2 2 2
  spline S63 degree 2 poles (-18.5023, 71.1843) (-18.4208, 71.0608) (-18.1392, 70.9349) (-17.9367, 70.9349) knots 0 0 0 1 2 2 2
  spline S64 degree 2 poles (-17.9367, 70.9349) (-17.7465, 70.9349) (-17.4501, 71.0608) (-17.3686, 71.1843) knots 0 0 0 1 2 2 2
  spline S65 degree 2 poles (-17.3686, 71.1843) (-17.292, 71.3004) (-17.2376, 71.5845) (-17.2376, 71.7895) knots 0 0 0 1 2 2 2
  line L69 (-17.2376, 71.7895) -> (-17.2376, 73.7013)
  line L70 (-17.2376, 73.7013) -> (-16.8326, 73.7013)
  line L71 (-16.8326, 73.7013) -> (-16.8326, 71.7994)
  spline S66 degree 2 poles (-16.8326, 71.7994) (-16.8326, 71.4807) (-16.961, 71.0263) (-17.124, 70.8706) knots 0 0 0 1 2 2 2
  spline S67 degree 2 poles (-17.124, 70.8706) (-17.2698, 70.7274) (-17.6551, 70.5891) (-17.9367, 70.5891) knots 0 0 0 1 2 2 2
  line L72 (-14.4861, 70.6533) -> (-14.8714, 70.6533)
  line L73 (-14.8714, 70.6533) -> (-14.8714, 71.9575)
  spline S68 degree 2 poles (-14.8714, 71.9575) (-14.8714, 72.1155) (-14.901, 72.3872) (-14.9455, 72.4687) knots 0 0 0 1 2 2 2
  spline S69 degree 2 poles (-14.9455, 72.4687) (-14.9924, 72.5552) (-15.1604, 72.6392) (-15.3036, 72.6392) knots 0 0 0 1 2 2 2
  spline S70 degree 2 poles (-15.3036, 72.6392) (-15.4469, 72.6392) (-15.7507, 72.486) (-15.8964, 72.3625) knots 0 0 0 1 2 2 2
  line L74 (-15.8964, 72.3625) -> (-15.8964, 70.6533)
  line L75 (-15.8964, 70.6533) -> (-16.2818, 70.6533)
  line L76 (-16.2818, 70.6533) -> (-16.2818, 72.9405)
  line L77 (-16.2818, 72.9405) -> (-15.8964, 72.9405)
  line L78 (-15.8964, 72.9405) -> (-15.8964, 72.6861)
  spline S71 degree 2 poles (-15.8964, 72.6861) (-15.7235, 72.8417) (-15.3901, 73.0047) (-15.2024, 73.0047) knots 0 0 0 1 2 2 2
  spline S72 degree 2 poles (-15.2024, 73.0047) (-14.8664, 73.0047) (-14.4861, 72.5601) (-14.4861, 72.1378) knots 0 0 0 1 2 2 2
  line L79 (-14.4861, 72.1378) -> (-14.4861, 70.6533)
  line L80 (-13.5524, 70.6533) -> (-13.9377, 70.6533)
  line L81 (-13.9377, 70.6533) -> (-13.9377, 72.9405)
  line L82 (-13.9377, 72.9405) -> (-13.5524, 72.9405)
  line L83 (-13.5524, 72.9405) -> (-13.5524, 70.6533)
  line L84 (-13.5252, 73.3209) -> (-13.9624, 73.3209)
  line L85 (-13.9624, 73.3209) -> (-13.9624, 73.721)
  line L86 (-13.9624, 73.721) -> (-13.5252, 73.721)
  line L87 (-13.5252, 73.721) -> (-13.5252, 73.3209)
  spline S73 degree 2 poles (-12.2951, 70.6088) (-12.6088, 70.6088) (-12.9621, 70.967) (-12.9621, 71.3548) knots 0 0 0 1 2 2 2
  line L88 (-12.9621, 71.3548) -> (-12.9621, 72.6219)
  line L89 (-12.9621, 72.6219) -> (-13.2214, 72.6219)
  line L90 (-13.2214, 72.6219) -> (-13.2214, 72.9405)
  line L91 (-13.2214, 72.9405) -> (-12.9621, 72.9405)
  line L92 (-12.9621, 72.9405) -> (-12.9621, 73.5975)
  line L93 (-12.9621, 73.5975) -> (-12.5767, 73.5975)
  line L94 (-12.5767, 73.5975) -> (-12.5767, 72.9405)
  line L95 (-12.5767, 72.9405) -> (-11.8678, 72.9405)
  line L96 (-11.8678, 72.9405) -> (-11.8678, 72.6219)
  line L97 (-11.8678, 72.6219) -> (-12.5767, 72.6219)
  line L98 (-12.5767, 72.6219) -> (-12.5767, 71.5326)
  spline S74 degree 2 poles (-12.5767, 71.5326) (-12.5767, 71.3597) (-12.5644, 71.1695) (-12.5224, 71.088) knots 0 0 0 1 2 2 2
  spline S75 degree 2 poles (-12.5224, 71.088) (-12.4878, 71.0164) (-12.3322, 70.9447) (-12.1988, 70.9447) knots 0 0 0 1 2 2 2
  spline S76 degree 2 poles (-12.1988, 70.9447) (-12.105, 70.9447) (-11.9296, 71.0016) (-11.8901, 71.0188) knots 0 0 0 1 2 2 2
  line L99 (-11.8901, 71.0188) -> (-11.8678, 71.0188)
  line L100 (-11.8678, 71.0188) -> (-11.8678, 70.673)
  spline S77 degree 2 poles (-11.8678, 70.673) (-11.9765, 70.6434) (-12.1988, 70.6088) (-12.2951, 70.6088) knots 0 0 0 1 2 2 2
  spline S78 degree 2 poles (-8.4345, 72.1773) (-8.4345, 71.3572) (-8.9112, 70.5891) (-9.4077, 70.5891) knots 0 0 0 1 2 2 2
  spline S79 degree 2 poles (-9.4077, 70.5891) (-9.9116, 70.5891) (-10.3834, 71.3721) (-10.3834, 72.1748) knots 0 0 0 1 2 2 2
  spline S80 degree 2 poles (-10.3834, 72.1748) (-10.3834, 72.9998) (-9.9066, 73.763) (-9.4077, 73.763) knots 0 0 0 1 2 2 2
  spline S81 degree 2 poles (-9.4077, 73.763) (-8.9063, 73.763) (-8.4345, 72.9726) (-8.4345, 72.1773) knots 0 0 0 1 2 2 2
  spline S82 degree 2 poles (-8.9582, 71.2486) (-8.8989, 71.3992) (-8.8495, 71.8636) (-8.8495, 72.1773) knots 0 0 0 1 2 2 2
  spline S83 degree 2 poles (-8.8495, 72.1773) (-8.8495, 72.491) (-8.8989, 72.9529) (-8.9606, 73.1085) knots 0 0 0 1 2 2 2
  spline S84 degree 2 poles (-8.9606, 73.1085) (-9.0224, 73.2641) (-9.2373, 73.4246) (-9.4077, 73.4246) knots 0 0 0 1 2 2 2
  spline S85 degree 2 poles (-9.4077, 73.4246) (-9.5781, 73.4246) (-9.798, 73.2641) (-9.8622, 73.1035) knots 0 0 0 1 2 2 2
  spline S86 degree 2 poles (-9.8622, 73.1035) (-9.9239, 72.9479) (-9.9684, 72.4737) (-9.9684, 72.1748) knots 0 0 0 1 2 2 2
  spline S87 degree 2 poles (-9.9684, 72.1748) (-9.9684, 71.8537) (-9.9289, 71.4239) (-9.8647, 71.256) knots 0 0 0 1 2 2 2
  spline S88 degree 2 poles (-9.8647, 71.256) (-9.8054, 71.0979) (-9.5855, 70.9275) (-9.4077, 70.9275) knots 0 0 0 1 2 2 2
  spline S89 degree 2 poles (-9.4077, 70.9275) (-9.2397, 70.9275) (-9.0199, 71.088) (-8.9582, 71.2486) knots 0 0 0 1 2 2 2
  line L101 (-6.1646, 70.6533) -> (-8.0442, 70.6533)
  line L102 (-8.0442, 70.6533) -> (-8.0442, 71.0855)
  spline S90 degree 2 poles (-8.0442, 71.0855) (-7.8417, 71.2757) (-7.4811, 71.6289) (-7.3082, 71.8191) knots 0 0 0 1 2 2 2
  spline S91 degree 2 poles (-7.3082, 71.8191) (-6.9599, 72.202) (-6.7055, 72.6614) (-6.7055, 72.9059) knots 0 0 0 1 2 2 2
  spline S92 degree 2 poles (-6.7055, 72.9059) (-6.7055, 73.0344) (-6.7845, 73.227) (-6.8562, 73.2888) knots 0 0 0 1 2 2 2
  spline S93 degree 2 poles (-6.8562, 73.2888) (-6.9278, 73.3505) (-7.1155, 73.4123) (-7.2291, 73.4123) knots 0 0 0 1 2 2 2
  spline S94 degree 2 poles (-7.2291, 73.4123) (-7.3378, 73.4123) (-7.5601, 73.358) (-7.6614, 73.316) knots 0 0 0 1 2 2 2
  spline S95 degree 2 poles (-7.6614, 73.316) (-7.7478, 73.2814) (-7.9084, 73.1826) (-7.9578, 73.148) knots 0 0 0 1 2 2 2
  line L103 (-7.9578, 73.148) -> (-7.98, 73.148)
  line L104 (-7.98, 73.148) -> (-7.98, 73.5827)
  spline S96 degree 2 poles (-7.98, 73.5827) (-7.8541, 73.6445) (-7.402, 73.7655) (-7.1995, 73.7655) knots 0 0 0 1 2 2 2
  spline S97 degree 2 poles (-7.1995, 73.7655) (-6.7722, 73.7655) (-6.2905, 73.3135) (-6.2905, 72.9282) knots 0 0 0 1 2 2 2
  spline S98 degree 2 poles (-6.2905, 72.9282) (-6.2905, 72.7479) (-6.3745, 72.4465) (-6.4486, 72.3181) knots 0 0 0 1 2 2 2
  spline S99 degree 2 poles (-6.4486, 72.3181) (-6.5227, 72.1847) (-6.7376, 71.9229) (-6.8562, 71.7969) knots 0 0 0 1 2 2 2
  spline S100 degree 2 poles (-6.8562, 71.7969) (-7.0488, 71.587) (-7.5206, 71.1374) (-7.6614, 71.0065) knots 0 0 0 1 2 2 2
  line L105 (-7.6614, 71.0065) -> (-6.1646, 71.0065)
  line L106 (-6.1646, 71.0065) -> (-6.1646, 70.6533)
  line L107 (-88.5815, 70.7891) -> (-88.5815, 73.4765)
  line L108 (-88.5815, 73.4765) -> (-89.6041, 73.4765)
  line L109 (-89.6041, 73.4765) -> (-89.6041, 73.8371)
  line L110 (-89.6041, 73.8371) -> (-87.1538, 73.8371)
  line L111 (-87.1538, 73.8371) -> (-87.1538, 73.4765)
  line L112 (-87.1538, 73.4765) -> (-88.1764, 73.4765)
  line L113 (-88.1764, 73.4765) -> (-88.1764, 70.7891)
  line L114 (-88.1764, 70.7891) -> (-88.5815, 70.7891)
  spline S101 degree 2 poles (-85.8818, 70.7373) (-86.4301, 70.7373) (-87.0328, 71.3523) (-87.0328, 71.9204) knots 0 0 0 1 2 2 2
  spline S102 degree 2 poles (-87.0328, 71.9204) (-87.0328, 72.4786) (-86.4474, 73.1406) (-85.9756, 73.1406) knots 0 0 0 1 2 2 2
  spline S103 degree 2 poles (-85.9756, 73.1406) (-85.7632, 73.1406) (-85.4347, 73.0171) (-85.3137, 72.8862) knots 0 0 0 1 2 2 2
  spline S104 degree 2 poles (-85.3137, 72.8862) (-85.1902, 72.7553) (-85.0592, 72.3774) (-85.0592, 72.1032) knots 0 0 0 1 2 2 2
  line L115 (-85.0592, 72.1032) -> (-85.0592, 71.8932)
  line L116 (-85.0592, 71.8932) -> (-86.6425, 71.8932)
  spline S105 degree 2 poles (-86.6425, 71.8932) (-86.6425, 71.4956) (-86.2424, 71.0732) (-85.8867, 71.0732) knots 0 0 0 1 2 2 2
  spline S106 degree 2 poles (-85.8867, 71.0732) (-85.7607, 71.0732) (-85.5162, 71.13) (-85.4174, 71.1745) knots 0 0 0 1 2 2 2
  spline S107 degree 2 poles (-85.4174, 71.1745) (-85.3137, 71.2239) (-85.1704, 71.3103) (-85.1235, 71.3498) knots 0 0 0 1 2 2 2
  line L117 (-85.1235, 71.3498) -> (-85.1012, 71.3498)
  line L118 (-85.1012, 71.3498) -> (-85.1012, 70.9299)
  spline S108 degree 2 poles (-85.1012, 70.9299) (-85.1679, 70.9028) (-85.3705, 70.8237) (-85.4495, 70.8015) knots 0 0 0 1 2 2 2
  spline S109 degree 2 poles (-85.4495, 70.8015) (-85.5607, 70.7694) (-85.7434, 70.7373) (-85.8818, 70.7373) knots 0 0 0 1 2 2 2
  spline S110 degree 2 poles (-85.4347, 72.1872) (-85.4396, 72.3428) (-85.5038, 72.57) (-85.5656, 72.6466) knots 0 0 0 1 2 2 2
  spline S111 degree 2 poles (-85.5656, 72.6466) (-85.6323, 72.733) (-85.8422, 72.8244) (-85.9979, 72.8244) knots 0 0 0 1 2 2 2
  spline S112 degree 2 poles (-85.9979, 72.8244) (-86.151, 72.8244) (-86.3659, 72.733) (-86.4548, 72.6441) knots 0 0 0 1 2 2 2
  spline S113 degree 2 poles (-86.4548, 72.6441) (-86.5413, 72.5527) (-86.6302, 72.3329) (-86.6425, 72.1872) knots 0 0 0 1 2 2 2
  line L119 (-86.6425, 72.1872) -> (-85.4347, 72.1872)